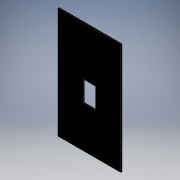
# Autodesk Inventor part: BA03
Saved by Autodesk Inventor 2017 (Build 210142000, 142)
## iProperties
Created: 2018-10-18
Part Number: BA03
Material: ABS Plastic
Document SubType Name: Modeling
Designer: Dell
Density: 1.06 g/cm^3
Appearance: Smooth - Black
Author: Dell
Autodesk Inventor part; units mm, degrees
ref_plane "YZ Plane" through (0, 0, 0) normal (1, 0, 0) x (0, 1, 0)
ref_plane "XZ Plane" through (0, 0, 0) normal (0, 1, 0) x (-1, 0, 0)
ref_plane "XY Plane" through (0, 0, 0) normal (0, 0, 1) x (1, 0, 0)
sketch "Sketch1" plane through (0, 0, 0) normal (0, 0, 1) x (1, 0, 0)
  line L0 (0, 0) -> (303.5592, 0)
  line L1 (303.5592, 0) -> (303.5592, -533.4)
  line L2 (303.5592, -533.4) -> (0, -533.4)
  line L3 (0, -533.4) -> (0, 0)
  line L4 (455.3388, 262.89) -> (303.5592, 0)
  line L5 (303.5592, 0) -> (0, 0)
  line L6 (0, 0) -> (-151.7796, 262.89)
  line L7 (-151.7796, 262.89) -> (0, 525.78)
  line L8 (0, 525.78) -> (303.5592, 525.78)
  line L9 (303.5592, 525.78) -> (455.3388, 262.89)
  point P0 (151.7796, 262.89)
  dimension "d1" = 533.4
  dimension "d54" = 525.78
  constraints: 20 end point, 2 parallel, 1 horizontal, 1 perpendicular, 13 other
  measures "d1" distance of L0.end L1.end
  measures "d54" distance between parallel lines of L7 L4
extrude "Extrusion1" add sketch "Sketch1" along normal blind 6.35 contours L0 L1 L2 L3
sketch "Sketch2" plane through (0, 0, 0) normal (0, 1, 0) x (1, 0, 0)
  line L0 (303.5592, -6.35) -> (0, -6.35) projected
  line L1 (0, -6.35) -> (-3.6662, -6.35)
  line L2 (-3.6662, -6.35) -> (0, 0)
  line L3 (0, 0) -> (0, -6.35) projected
  line L4 (0, 0) -> (0, -6.35) projected
  line L5 (0, -6.35) -> (0, 0)
  line L6 (303.5592, -6.35) -> (307.2254, -6.35)
  line L7 (303.5592, 0) -> (303.5592, -6.35) projected
  line L8 (307.2254, -6.35) -> (303.5592, 0)
  line L9 (303.5592, 0) -> (303.5592, -6.35)
  dimension "d4" = 30
  dimension "d5" = 60
  constraints: 12 end point, 2 collinear, 2 horizontal
  measures "d4" angle of L3 L2
  measures "d5" angle of L6 L8
extrude "Extrusion2" add sketch "Sketch2" against normal blind 533.4
sketch "Sketch4" plane through (0, 0, 6.35) normal (0, 0, 1) x (1, 0, 0)
  line L0 (137.7796, -228.6) -> (165.7796, -228.6)
  line L1 (165.7796, -228.6) -> (165.7796, -278.6)
  line L2 (165.7796, -278.6) -> (137.7796, -278.6)
  line L3 (137.7796, -278.6) -> (137.7796, -228.6)
  line L4 (-3.6662, 0) -> (-3.6662, -533.4) projected
  line L5 (-3.6662, 0) -> (307.2254, 0) projected
  line L6 (307.2254, -533.4) -> (-3.6662, -533.4) projected
  circle A0 centre (131.7796, -253.6) radius 3
  circle A1 centre (171.7796, -253.6) radius 3
  point P0 (0, 0)
  point P1 (151.7796, -228.6)
  point P2 (151.7796, 0)
  point P3 (165.7796, -253.6)
  point P4 (137.7796, -253.6)
  dimension "d16" = 28
  dimension "d17" = 50
  dimension "d19" = 6
  dimension "d20" = 6
  dimension "d21" = 6
  dimension "d22" = 6
  dimension "d41" = 228.6
  constraints: 8 end point, 4 midpoint, 2 centre point, 2 horizontal alignment, 2 parallel, 1 horizontal, 1 perpendicular, 1 vertical alignment
  measures "d16" distance of L1.end L2.end
  measures "d17" distance of L0.end L1.end
  measures "d19" diameter of A0
  measures "d20" diameter of A1
  measures "d21" distance from line of L3 A0.centre
  measures "d22" distance from line of A1.centre L1
  measures "d41" distance between parallel lines of L5 L0
extrude "Extrusion4" cut sketch "Sketch4" against normal through all
sketch "Sketch5" plane through (0, 0, 6.35) normal (0, 0, 1) x (1, 0, 0)
  line L0 (195.2796, -309.6) -> (108.2796, -309.6)
  line L1 (108.2796, -309.6) -> (108.2796, -298.6)
  line L2 (108.2796, -298.6) -> (195.2796, -298.6)
  line L3 (195.2796, -298.6) -> (195.2796, -309.6)
  line L4 (165.7796, -278.6) -> (137.7796, -278.6) projected
  line L5 (181.2796, -330.6) -> (159.2796, -330.6)
  line L6 (159.2796, -330.6) -> (159.2796, -318.6)
  line L7 (159.2796, -318.6) -> (181.2796, -318.6)
  line L8 (181.2796, -318.6) -> (181.2796, -330.6)
  line L9 (144.2796, -334.6) -> (122.2796, -334.6)
  line L10 (122.2796, -334.6) -> (122.2796, -314.6)
  line L11 (122.2796, -314.6) -> (144.2796, -314.6)
  line L12 (144.2796, -314.6) -> (144.2796, -334.6)
  line L13 (159.2796, -324.6) -> (144.2796, -324.6) construction
  point P0 (0, 0)
  point P1 (151.7796, -298.6)
  point P2 (151.7796, -278.6)
  point P3 (151.7796, -324.6)
  dimension "d26" = 87
  dimension "d27" = 11
  dimension "d28" = 20
  dimension "d29" = 22
  dimension "d30" = 12
  dimension "d32" = 22
  dimension "d33" = 20
  dimension "d37" = 15
  dimension "d38" = 15
  constraints: 26 end point, 6 parallel, 5 midpoint, 4 horizontal, 3 perpendicular, 2 vertical alignment, 1 horizontal alignment
  measures "d26" distance of L1.end L2.end
  measures "d27" distance of L0.end L1.end
  measures "d28" distance between parallel lines of L4 L2
  measures "d29" distance of L6.end L7.end
  measures "d30" distance of L5.end L6.end
  measures "d32" distance of L10.end L11.end
  measures "d33" distance of L9.end L10.end
  measures "d37" distance from line of L0 L13.start
  measures "d38" distance between parallel lines of L12 L6
extrude "Extrusion5" cut sketch "Sketch5" against normal through all
sketch "Sketch7" plane through (0, 0, 6.35) normal (0, 0, 1) x (1, 0, 0)
  line L0 (101.7796, -345) -> (201.7796, -345)
  line L1 (201.7796, -345) -> (201.7796, -225)
  line L2 (201.7796, -225) -> (101.7796, -225)
  line L3 (101.7796, -225) -> (101.7796, -345)
  line L4 (-3.6662, 0) -> (307.2254, 0) projected
  point P0 (0, 0)
  point P1 (151.7796, -225)
  point P2 (151.7796, 0)
  dimension "d49" = 100
  dimension "d50" = 120
  dimension "d51" = 225
  constraints: 8 end point, 2 midpoint, 2 parallel, 1 horizontal, 1 perpendicular, 1 vertical alignment
  measures "d49" distance of L1.end L2.end
  measures "d50" distance of L0.end L1.end
  measures "d51" distance between parallel lines of L4 L2
extrude "Extrusion7" cut sketch "Sketch7" against normal through all
sketch "Sketch8" plane through (0, 0, 0) normal (0, 1, 0) x (1, 0, 0)
  line L0 (-3.6662, -6.35) -> (307.2254, -6.35) projected
  line L1 (0, 0) -> (-3.6662, 0)
  line L2 (-3.6662, 0) -> (-3.6662, -6.35)
  line L3 (-3.6662, -6.35) -> (0, -6.35)
  line L4 (0, -6.35) -> (0, 0)
  line L5 (0, 0) -> (303.5592, 0) projected
  line L6 (307.2254, -6.35) -> (303.5592, -6.35)
  line L7 (303.5592, -6.35) -> (303.5592, 0)
  line L8 (303.5592, 0) -> (307.2254, 0)
  line L9 (307.2254, 0) -> (307.2254, -6.35)
  constraints: 16 end point, 4 parallel, 2 horizontal, 2 perpendicular
extrude "Extrusion8" cut sketch "Sketch8" against normal through all contours L2 L1 L4 L0 | L7 L8 L9 L0
sketch "Sketch9" plane through (0, 0, 6.35) normal (0, 0, 1) x (1, 0, 0)
  line L0 (121.7796, -335) -> (181.7796, -335)
  line L1 (181.7796, -335) -> (181.7796, -235)
  line L2 (181.7796, -235) -> (121.7796, -235)
  line L3 (121.7796, -235) -> (121.7796, -335)
  line L4 (0, 0) -> (303.5592, 0) projected
  line L5 (101.7796, -345) -> (101.7796, -225) projected
  line L6 (201.7796, -225) -> (201.7796, -345) projected
  line L7 (201.7796, -345) -> (101.7796, -345) projected
  line L8 (101.7796, -345) -> (101.7796, -225) projected
  line L9 (101.7796, -225) -> (201.7796, -225) projected
  line L10 (0, 0) -> (0, -533.4) projected
  line L11 (303.5592, -533.4) -> (0, -533.4) projected
  line L12 (303.5592, -533.4) -> (303.5592, 0) projected
  line L13 (0, 0) -> (303.5592, 0) projected
  point P0 (121.7796, -285)
  point P1 (101.7796, -285)
  point P2 (151.7796, -235)
  point P3 (151.7796, 0)
  dimension "d57" = 60
  dimension "d58" = 100
  constraints: 8 end point, 4 midpoint, 2 parallel, 1 horizontal, 1 horizontal alignment, 1 perpendicular, 1 vertical alignment
  measures "d57" distance of L1.end L2.end
  measures "d58" distance of L0.end L1.end
extrude "Extrusion9" add sketch "Sketch9" against normal blind 6.35 contours L5 L9 L6 L7
body "Solid1"
